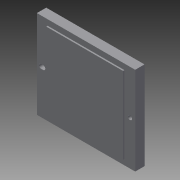
# Autodesk Inventor part: KAC12040
Saved by Autodesk Inventor 2013 (Build 170138000, 138)
## iProperties
Created: 2014-04-26
Part Number: KAC12040
Material: Generic
Document SubType Name: Modeling
Designer: spichelh
Density: 1 g/cm^3
Author: spichelh
Autodesk Inventor part; units mm, degrees
ref_plane "YZ Plane" through (0, 0, 0) normal (1, 0, 0) x (0, 1, 0)
ref_plane "XZ Plane" through (0, 0, 0) normal (0, 1, 0) x (-1, 0, 0)
ref_plane "XY Plane" through (0, 0, 0) normal (0, 0, 1) x (1, 0, 0)
sketch "Sketch1" plane through (0, 0, 0) normal (0, 0, 1) x (1, 0, 0)
  line L0 (-21.25, 19.05) -> (21.25, 19.05)
  line L1 (21.25, 19.05) -> (21.25, -19.05)
  line L2 (21.25, -19.05) -> (-21.25, -19.05)
  line L3 (-21.25, -19.05) -> (-21.25, 19.05)
  line L4 (21.25, 0) -> (-21.25, 0) construction
  circle A0 centre (19, 0) radius 0.875
  line L5 (-19.445, 0.915) -> (-18.555, 0.915)
  line L6 (-18.555, -0.915) -> (-19.445, -0.915)
  arc A1 (-19.445, 0.915) -> (-19.445, -0.915) centre (-19.445, 0) ccw
  arc A2 (-18.555, -0.915) -> (-18.555, 0.915) centre (-18.555, 0) ccw
  line L7 (0, -19.05) -> (0, 19.05) construction
  line L8 (-19, 0.915) -> (-19, -0.915) construction
  point P0 (0, 0)
  point P1 (-19, 0)
  dimension "d0" = 38.1
  dimension "d2" = 42.5
  dimension "d3" = 2.25
  dimension "d4" = 1.75
  dimension "d6" = 1.83
  dimension "d7" = 2.72
  dimension "d8" = 38
  constraints: 18 end point, 9 midpoint, 4 point on circle, 4 tangent, 3 centre point, 3 parallel, 2 horizontal, 2 point on line, 1 perpendicular
  measures "d0" distance of L2.end L0.start
  measures "d2" distance of L0.start L0.end
  measures "d3" distance from line of L1 A0.centre
  measures "d4" diameter of A0
  measures "d6" distance between parallel lines of L5 L6
  measures "d8" distance of point (-19, 0) A0.centre
extrude "Extrusion1" add sketch "Sketch1" along normal blind 4.04
sketch "Sketch2" plane through (0, 0, 4.04) normal (0, 0, 1) x (1, 0, 0)
  line L0 (-16.61, 16.61) -> (16.61, 16.61)
  line L1 (16.61, 16.61) -> (16.61, -16.61)
  line L2 (16.61, -16.61) -> (-16.61, -16.61)
  line L3 (-16.61, -16.61) -> (-16.61, 16.61)
  line L4 (0, 16.61) -> (0, -16.61) construction
  line L5 (-16.61, 0) -> (16.61, 0) construction
  point P0 (0, 0)
  dimension "d11" = 33.22
  dimension "d18" = 33.22
  constraints: 12 end point, 6 midpoint, 2 parallel, 1 horizontal, 1 perpendicular
  measures "d11" distance of L0.start L0.end
  measures "d18" distance between parallel lines of L0 L2
extrude "Extrusion2" add sketch "Sketch2" along normal blind 0.61
sketch "Sketch3" plane through (0, 0, 4.65) normal (0, 0, 1) x (1, 0, 0)
  line L0 (16.61, 16.61) -> (-16.61, 16.61) projected
  line L1 (-16.61, 16.61) -> (-16.61, -16.61) projected
  line L2 (-16.61, -16.61) -> (16.61, -16.61) projected
  line L3 (16.61, -16.61) -> (16.61, 16.61) projected
  line L4 (-9.5505, 7.125) -> (9.5505, 7.125)
  line L5 (9.5505, 7.125) -> (9.5505, -7.125)
  line L6 (9.5505, -7.125) -> (-9.5505, -7.125)
  line L7 (-9.5505, -7.125) -> (-9.5505, 7.125)
  line L8 (-9.5505, 7.125) -> (9.5505, -7.125) construction
  line L9 (9.5505, 7.125) -> (-9.5505, -7.125) construction
  point P0 (0, 0)
  point P1 (0, 0)
  dimension "d21" = 19.101
  dimension "d23" = 14.25
  constraints: 12 end point, 2 midpoint, 2 parallel, 1 coincident, 1 horizontal, 1 perpendicular
  measures "d21" distance of L4.start L4.end
  measures "d23" distance of L6.end L4.start
body "Solid1"
